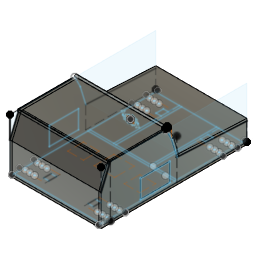
structure_vistech006_vigorini v10 (Autodesk Fusion 360 design; units mm, degrees)
Autodesk Fusion 360 part; units mm, degrees
note: some values were not read from the file. Set by a fixed rule: which face or edge a step refers to.
sketch "Sketch1" plane through (0, 0, 0) normal (0, 0, 1) x (1, 0, 0) in component "Base"
  line L0 (-125, -200) -> (125, -200)
  line L1 (125, -200) -> (125, 200)
  line L2 (125, 200) -> (-125, 200)
  line L3 (-125, 200) -> (-125, -200)
  line L4 (-125, -200) -> (125, 200) construction
  line L5 (125, -200) -> (-125, 200) construction
  dimension "d1" = 250
  dimension "d2" = 400
  constraint horizontal L0
  constraint perpendicular L0 L1
  constraint parallel L0 L2
  constraint parallel L1 L3
  constraint coincident L4 origin
  constraint coincident L5 origin
  measures "d1" distance of L1.end L2.end
  measures "d2" distance of L0.end L1.end
extrude "Extrude1" add sketch "Sketch1" along normal blind 6 makes body 1 in component "Base"
sketch "Sketch2" plane through (0, 0, 6) normal (0, 0, 1) x (-1, 0, 0) in component "Base"
  line L0 (125, -200) -> (125, 200)
  line L1 (125, 200) -> (-125, 200)
  line L2 (-125, 200) -> (-125, -200)
  line L3 (-125, -200) -> (125, -200)
  line L4 (-119, -194) -> (119, -194)
  line L5 (119, 194) -> (-119, 194)
  line L6 (-119, 194) -> (-119, -194)
  line L7 (119, 194) -> (119, -194)
  line L8 (-119, -194) -> (-119, -200)
  line L9 (119, -194) -> (119, -200)
  line L10 (-119, 194) -> (-119, 200)
  line L11 (119, 194) -> (119, 200)
  line L12 (-119, -194) -> (-119, -14) construction
  line L13 (-119, -14) -> (-119, 194) construction
  line L14 (-119, -14) -> (119, -14)
  line L15 (-93.6209, -8.2136) -> (-93.6209, -8) construction
  line L16 (-119, -8.2136) -> (119, -8.2136)
  line L17 (-48, -194) -> (-48, -14)
  line L18 (48, -194) -> (48, -14)
  line L19 (-125, -174) -> (-54, -174) construction
  line L20 (-54, -174) -> (-54, -164) construction
  line L21 (-54, -164) -> (-68.1, -164)
  line L22 (-68.1, -164) -> (-68.1, -144)
  line L23 (-68.1, -144) -> (-54, -144)
  line L24 (-54, -144) -> (-54, -134) construction
  line L25 (-54, -134) -> (-125, -134) construction
  line L26 (-54, -194) -> (-54, -14)
  line L27 (125, -174) -> (54, -174) construction
  line L28 (54, -174) -> (54, -164) construction
  line L29 (54, -164) -> (68.1, -164)
  line L30 (68.1, -164) -> (68.1, -144)
  line L31 (68.1, -144) -> (54, -144)
  line L32 (54, -144) -> (54, -134) construction
  line L33 (54, -134) -> (125, -134) construction
  line L34 (54.2628, -194) -> (54.2628, -14)
  line L35 (125, 174) -> (54, 174) construction
  line L36 (54, 174) -> (54, 164) construction
  line L37 (54, 164) -> (68.1, 164)
  line L38 (68.1, 164) -> (68.1, 144)
  line L39 (68.1, 144) -> (54, 144)
  line L40 (54, 144) -> (54, 134) construction
  line L41 (54, 134) -> (125, 134) construction
  line L42 (-125, 174) -> (-54, 174) construction
  line L43 (-54, 174) -> (-54, 164) construction
  line L44 (-54, 164) -> (-68.1, 164)
  line L45 (-68.1, 164) -> (-68.1, 144)
  line L46 (-68.1, 144) -> (-54, 144)
  line L47 (-54, 144) -> (-54, 134) construction
  line L48 (-54, 134) -> (-125, 134) construction
  circle A0 centre (-112.12, -137.2) radius 1.5
  circle A1 centre (-99.32, -137.2) radius 1.5
  circle A2 centre (-86.52, -137.2) radius 1.5
  circle A3 centre (-112.2, -170.8) radius 1.5
  circle A4 centre (-99.4, -170.8) radius 1.5
  circle A5 centre (-86.6, -170.8) radius 1.5
  circle A6 centre (112.2, -137.2) radius 1.5
  circle A7 centre (99.4, -137.2) radius 1.5
  circle A8 centre (86.6, -137.2) radius 1.5
  circle A9 centre (86.6, -170.8) radius 1.5
  circle A10 centre (112.2, -170.8) radius 1.5
  circle A11 centre (99.4, -170.8) radius 1.5
  circle A12 centre (-112.2, 137.2) radius 1.5
  circle A13 centre (-99.4, 137.2) radius 1.5
  circle A14 centre (-86.6, 137.2) radius 1.5
  circle A15 centre (-112.2, 170.8) radius 1.5
  circle A16 centre (-99.4, 170.8) radius 1.5
  circle A17 centre (-86.6, 170.8) radius 1.5
  circle A18 centre (112.2, 170.8) radius 1.5
  circle A19 centre (99.4, 170.8) radius 1.5
  circle A20 centre (86.6, 170.8) radius 1.5
  circle A21 centre (112.2, 137.2) radius 1.5
  circle A22 centre (99.4, 137.2) radius 1.5
  circle A23 centre (86.6, 137.2) radius 1.5
  line L49 (54, 144) -> (54, 164)
  line L50 (-54, 144) -> (-54, 164)
  line L51 (28.025, 11.7864) -> (28.025, 65.8664) construction
  line L52 (28.025, 65.8664) -> (-28.025, 65.8664) construction
  line L53 (-28.025, 65.8664) -> (-28.025, 61.3869) construction
  line L54 (-28.025, 61.3869) -> (-28.025, 11.7864) construction
  line L55 (-28.025, 11.7864) -> (28.025, 11.7864) construction
  line L56 (-99, 24.3105) -> (-56, 24.3105) construction
  line L57 (-56, 24.3105) -> (-56, 67.5105) construction
  line L58 (-56, 67.5105) -> (-99, 67.5105) construction
  line L59 (-99, 67.5105) -> (-99, 24.3105) construction
  line L60 (99, 24.3105) -> (99, 67.5105) construction
  line L61 (99, 67.5105) -> (56, 67.5105) construction
  line L62 (56, 67.5105) -> (56, 24.3105) construction
  line L63 (56, 24.3105) -> (99, 24.3105) construction
  dimension "d9" = 388
  dimension "d10" = 238
  dimension "d11" = 180
  dimension "d14" = 202.2136
  dimension "d18" = 71
  dimension "d21" = 20
  dimension "d22" = 14.1
  dimension "d23" = 10
  dimension "d25" = 71
  dimension "d28" = 20
  dimension "d29" = 14.1
  dimension "d32" = 71
  dimension "d33" = 10
  dimension "d34" = 14.1
  dimension "d35" = 20
  dimension "d39" = 71
  dimension "d40" = 10
  dimension "d41" = 14.1
  dimension "d42" = 20
  dimension "d53" = 12.8
  dimension "d54" = 12.8
  dimension "d58" = 3
  dimension "d59" = 3
  dimension "d60" = 3
  dimension "d61" = 3
  dimension "d62" = 3
  dimension "d63" = 3
  dimension "d68" = 12.8
  dimension "d70" = 3
  dimension "d71" = 3
  dimension "d72" = 3
  dimension "d73" = 3
  dimension "d74" = 3
  dimension "d75" = 3
  dimension "d79" = 12.8
  dimension "d80" = 12.8
  dimension "d85" = 3
  dimension "d86" = 3
  dimension "d87" = 3
  dimension "d88" = 3
  dimension "d89" = 3
  dimension "d90" = 3
  dimension "d94" = 12.8
  dimension "d95" = 12.8
  dimension "d100" = 3
  dimension "d101" = 3
  dimension "d102" = 3
  dimension "d109" = 12.8
  dimension "d110" = 3
  dimension "d111" = 3
  dimension "d112" = 3
  dimension "d115" = 54.08
  dimension "d116" = 56.05
  dimension "d118" = 43
  dimension "d119" = 43.2
  dimension "d121" = 43.2
  dimension "d122" = 43
  constraint perpendicular L0 L4
  constraint perpendicular L2 L5
  constraint perpendicular L3 L6
  constraint perpendicular L3 L7
  constraint coincident L3 L8.end
  constraint perpendicular L3 L8
  constraint coincident L3 L9.end
  constraint perpendicular L3 L9
  constraint coincident L1 L10.end
  constraint perpendicular L1 L10
  constraint coincident L1 L11.end
  constraint perpendicular L1 L11
  constraint perpendicular L4 L12
  constraint perpendicular L5 L13
  constraint coincident L7 L14.end
  constraint perpendicular L7 L14
  constraint perpendicular L14 L15
  constraint coincident L6 L16.start
  constraint coincident L7 L16.end
  constraint perpendicular L7 L16
  constraint coincident L16 L15.start
  constraint coincident L4 L17.start
  constraint coincident L14 L17.end
  constraint perpendicular L14 L17
  constraint coincident L4 L18.start
  constraint coincident L14 L18.end
  constraint perpendicular L14 L18
  constraint coincident L2 L19.start
  constraint perpendicular L2 L19
  constraint perpendicular L19 L20
  constraint perpendicular L20 L21
  constraint perpendicular L21 L22
  constraint perpendicular L22 L23
  constraint perpendicular L23 L24
  constraint coincident L2 L25.end
  constraint perpendicular L2 L25
  constraint coincident L4 L26.start
  constraint perpendicular L14 L26
  constraint coincident L0 L27.start
  constraint perpendicular L7 L27
  constraint perpendicular L27 L28
  constraint perpendicular L28 L29
  constraint perpendicular L29 L30
  constraint perpendicular L30 L31
  constraint perpendicular L31 L32
  constraint coincident L0 L33.end
  constraint perpendicular L0 L33
  constraint coincident L4 L34.start
  constraint coincident L14 L34.end
  constraint perpendicular L14 L34
  constraint coincident L0 L35.start
  constraint perpendicular L34 L35
  constraint perpendicular L35 L36
  constraint perpendicular L34 L37
  constraint perpendicular L16 L38
  constraint perpendicular L38 L39
  constraint perpendicular L39 L40
  constraint coincident L0 L41.end
  constraint perpendicular L0 L41
  constraint coincident L2 L42.start
  constraint perpendicular L13 L42
  constraint perpendicular L42 L43
  constraint perpendicular L43 L44
  constraint perpendicular L44 L45
  constraint perpendicular L45 L46
  constraint perpendicular L46 L47
  constraint coincident L2 L48.end
  constraint perpendicular L2 L48
  constraint perpendicular L37 L49
  constraint perpendicular L44 L50
  constraint perpendicular L51 L52
  constraint perpendicular L52 L53
  constraint perpendicular L52 L54
  constraint perpendicular L51 L55
  constraint perpendicular L56 L57
  constraint perpendicular L56 L59
  constraint perpendicular L60 L61
  constraint perpendicular L61 L62
  constraint perpendicular L60 L63
  measures "d9" distance of L4.start L5.end
  measures "d10" distance of L5.start L5.end
  measures "d11" distance of L4.start L12.end
  measures "d14" distance of L5.end L16.start
  measures "d18" distance of L19.start L19.end
  measures "d21" distance of L21.end L22.end
  measures "d22" distance of L22.end L23.end
  measures "d23" distance of L23.end L24.end
  measures "d25" distance of L27.start L27.end
  measures "d28" distance of L29.end L30.end
  measures "d29" distance of L30.end L31.end
  measures "d32" distance of L35.start L35.end
  measures "d33" distance of L35.end L36.end
  measures "d34" distance of L36.end L37.end
  measures "d35" distance of L37.end L38.end
  measures "d39" distance of L42.start L42.end
  measures "d40" distance of L42.end L43.end
  measures "d41" distance of L43.end L44.end
  measures "d42" distance of L44.end L45.end
  measures "d53" distance of A0.centre A1.centre
  measures "d54" distance of A1.centre A2.centre
  measures "d58" diameter of A0
  measures "d59" diameter of A1
  measures "d60" diameter of A2
  measures "d61" diameter of A3
  measures "d62" diameter of A4
  measures "d63" diameter of A5
  measures "d68" distance of A7.centre A8.centre
  measures "d70" diameter of A8
  measures "d71" diameter of A7
  measures "d72" diameter of A6
  measures "d73" diameter of A9
  measures "d74" diameter of A11
  measures "d75" diameter of A10
  measures "d79" distance of A15.centre A16.centre
  measures "d80" distance of A16.centre A17.centre
  measures "d85" diameter of A12
  measures "d86" diameter of A13
  measures "d87" diameter of A14
  measures "d88" diameter of A15
  measures "d89" diameter of A16
  measures "d90" diameter of A17
  measures "d94" distance of A18.centre A19.centre
  measures "d95" distance of A19.centre A20.centre
  measures "d100" diameter of A20
  measures "d101" diameter of A19
  measures "d102" diameter of A18
  measures "d109" distance of A22.centre A23.centre
  measures "d110" diameter of A23
  measures "d111" diameter of A22
  measures "d112" diameter of A21
  measures "d115" distance of L51.start L51.end
  measures "d116" distance of L51.end L52.end
  measures "d118" distance of L56.start L56.end
  measures "d119" distance of L56.end L57.end
  measures "d121" distance of L60.start L60.end
  measures "d122" distance of L60.end L61.end
extrude "Extrude2" cut sketch "Sketch2" along normal through all and the other way through all contours L29 L30 L31 L34 | L21 L22 L23 L26 | L37 L38 L39 L49 | L44 L45 L46 L50 | A0 | A1 | A2 | A3 | A4 | A5 | A6 | A7 | A8 | A9 | A10 | A11 | A12 | A13 | A14 | A15 | A16 | A17 | A18 | A19 | A20 | A21 | A22 | A23 bodies 1 in component "Base"
sketch "Sketch2 (2)" plane through (0, 0, 6) normal (0, 0, 1) x (-1, 0, 0) in component "Right_panel"
extrude "Extrude1'" add sketch "Sketch2" along normal blind 140 separate body contours L1 L2 L3 L6 L8 L10 makes body 2 in component "Right_panel"
sketch "Sketch3" plane through (125, 0, 0) normal (1, 0, 0) x (0, 1, 0) in component "Right_panel"
  line L0 (-200, 6) -> (200, 6)
  line L1 (200, 6) -> (200, 146)
  line L2 (200, 146) -> (-200, 146)
  line L3 (-200, 146) -> (-200, 6)
  line L4 (200, 6) -> (200, 56) construction
  line L5 (200, 6) -> (8, 6) construction
  line L6 (8, 6) -> (8, 66) construction
  line L7 (8, 66) -> (8, 116) construction
  line L8 (8, 66) -> (200, 56)
  line L9 (-7, 116) -> (8, 66)
  line L10 (-7, 116) -> (-22, 146)
  line L11 (-7, 116) -> (-7, 146) construction
  line L12 (-7, 146) -> (-22, 146) construction
  line L13 (-200, 146) -> (-200, 86) construction
  line L14 (-200, 146) -> (-175, 146) construction
  line L15 (-200, 86) -> (-175, 146)
  line L16 (-12, 66) -> (-92, 66)
  line L17 (-92, 66) -> (-92, 16)
  line L18 (-92, 16) -> (-12, 16)
  line L19 (-12, 16) -> (-12, 66)
  line L20 (-175, 146) -> (-175, 6) construction
  dimension "d152" = 50
  dimension "d153" = 192
  dimension "d155" = 60
  dimension "d156" = 50
  dimension "d157" = 15
  dimension "d159" = 30
  dimension "d160" = 15
  dimension "d161" = 60
  dimension "d162" = 25
  dimension "d164" = 20
  dimension "d165" = 80
  dimension "d166" = 50
  dimension "d167" = 140
  constraint coincident L0.end L1.start
  constraint perpendicular L0 L4
  constraint perpendicular L1 L5
  constraint perpendicular L5 L6
  constraint parallel L6 L7
  constraint coincident L2 L10.end
  constraint perpendicular L2 L11
  constraint perpendicular L11 L12
  constraint coincident L2.end L3.start
  constraint perpendicular L2 L13
  constraint perpendicular L3 L14
  constraint perpendicular L16 L17
  constraint perpendicular L17 L18
  constraint perpendicular L16 L19
  constraint perpendicular L0 L20
  measures "d152" distance of L0.end L4.end
  measures "d153" distance of L0.end L5.end
  measures "d155" distance of L5.end L6.end
  measures "d156" distance of L6.end L7.end
  measures "d157" distance of L7.end L9.start
  measures "d159" distance of L9.start L11.end
  measures "d160" distance of L11.end L10.end
  measures "d161" distance of L2.end L13.end
  measures "d162" distance of L2.end L14.end
  measures "d164" distance of L6.end L16.start
  measures "d165" distance of L16.start L16.end
  measures "d166" distance of L16.end L17.end
  measures "d167" distance of L14.end L20.end
extrude "Extrude2'" cut sketch "Sketch3" against normal through all contours L2 L3 L15 | L1 L2 L8 L9 L10 bodies 2 in component "Right_panel"
sketch "Sketch1 (2)" plane through (0, 0, 6) normal (0, 0, 1) x (-1, 0, 0) in component "left_panel"
extrude "Extrude1''" add sketch "Sketch2" along normal blind 140 separate body contours L0 L1 L3 L7 L9 L11 makes body 3 in component "left_panel"
sketch "Sketch2 (3)" plane through (-125, 0, 0) normal (-1, 0, 0) x (0, -1, 0) in component "left_panel"
  line L0 (-200, 6) -> (200, 6)
  line L1 (200, 6) -> (200, 146)
  line L2 (200, 146) -> (-200, 146)
  line L3 (-200, 146) -> (-200, 6)
  line L4 (-200, 6) -> (-8, 6) construction
  line L5 (-200, 6) -> (-200, 56) construction
  line L6 (-8, 6) -> (-8, 66) construction
  line L7 (-8, 66) -> (7, 116)
  line L8 (7, 116) -> (22, 146)
  line L9 (-8, 66) -> (-200, 56)
  line L10 (12, 66) -> (92, 66)
  line L11 (92, 66) -> (92, 16)
  line L12 (92, 16) -> (12, 16)
  line L13 (12, 16) -> (12, 66)
  line L14 (200, 146) -> (175, 146) construction
  line L15 (200, 146) -> (200, 86)
  line L16 (175, 146) -> (200, 86)
  dimension "d170" = 192
  dimension "d171" = 50
  dimension "d172" = 60
  dimension "d177" = 80
  dimension "d178" = 50
  dimension "d180" = 25
  dimension "d181" = 60
  constraint coincident L0.start L3.end
  constraint perpendicular L3 L4
  constraint perpendicular L4 L5
  constraint perpendicular L4 L6
  constraint perpendicular L10 L11
  constraint perpendicular L11 L12
  constraint coincident L1.end L2.start
  constraint perpendicular L1 L14
  constraint perpendicular L14 L15
  measures "d170" distance of L0.start L4.end
  measures "d171" distance of L0.start L5.end
  measures "d172" distance of L4.end L6.end
  measures "d177" distance of L10.start L10.end
  measures "d178" distance of L10.end L11.end
  measures "d180" distance of L1.end L14.end
  measures "d181" distance of L1.end L15.end
extrude "Extrude2''" cut sketch "Sketch2 (3)" against normal through all contours L2 L3 L7 L8 L9 | L1 L2 L15 L16 bodies 3 in component "left_panel"
extrude "Extrude4" cut sketch "Sketch2 (3)" against normal up to surface (6 mm away) contours L10 L11 L12 L13 bodies 3 in component "left_panel"
extrude "Extrude4'" cut sketch "Sketch3" against normal up to surface (6 mm away) contours L16 L17 L18 L19 bodies 2 in component "Right_panel"
sketch "Sketch1 (3)" plane through (125, 0, 0) normal (1, 0, 0) x (0, 1, 0) in component "Right_driver_panel"
extrude "Extrude1'''" add sketch "Sketch3" against normal up to surface (6 mm away) separate body contours L16 L17 L18 L19 makes body 4 in component "Right_driver_panel"
sketch "Sketch1 (4)" plane through (-125, 0, 0) normal (-1, 0, 0) x (0, -1, 0) in component "Left_driver_panel"
extrude "Extrude1''''" add sketch "Sketch2 (3)" against normal up to surface (6 mm away) separate body contours L10 L11 L12 L13 makes body 5 in component "Left_driver_panel"
sketch "Sketch1 (5)" plane through (0, 0, 6) normal (0, 0, 1) x (-1, 0, 0) in component "Front_panel"
extrude "Extrude1'''''" add sketch "Sketch2" along normal blind 50 separate body contours L3 L4 L8 L9 makes body 6 in component "Front_panel"
sketch "Sketch1 (6)" plane through (0, 0, 6) normal (0, 0, 1) x (-1, 0, 0) in component "mid_panel"
extrude "Extrude1''''''" add sketch "Sketch2" along normal blind 60 separate body contours L6 L7 L14 L16 makes body 7 in component "mid_panel"
extrude "Extrude1'''''''" add sketch "Sketch2" along normal blind 80 separate body contours L1 L5 L10 L11 makes body 8 in component "Back_panel"
extrude "Extrude1''''''''" add sketch "Sketch2" along normal blind 60 separate body contours L4 L14 L17 L26 makes body 9 in component "Front_support_right_panel"
sketch "Sketch1 (7)" plane through (48, 0, 0) normal (-1, 0, 0) x (0, -1, 0) in component "Front_support_right_panel"
  line L0 (-194, 6) -> (-14, 6)
  line L1 (-14, 6) -> (-14, 66)
  line L2 (-14, 66) -> (-194, 66)
  line L3 (-194, 66) -> (-194, 6)
  line L4 (-194, 66) -> (-194, 56) construction
  line L5 (-194, 56) -> (-14, 66)
  dimension "d203" = 10
  constraint coincident L2.end L3.start
  constraint perpendicular L2 L4
  constraint coincident L1.end L2.start
  measures "d203" distance of L2.end L4.end
extrude "Extrude2'''" cut sketch "Sketch1 (7)" against normal up to surface (6 mm away) contours L2 L3 L5 bodies 9 in component "Front_support_right_panel"
extrude "Extrude1'''''''''" add sketch "Sketch2" along normal blind 60 separate body contours L4 L14 L18 L34 makes body 10 in component "Front_support_left_panel"
sketch "Sketch1 (8)" plane through (-54.2628, 0, 0) normal (-1, 0, 0) x (0, -1, 0) in component "Front_support_left_panel"
  line L0 (-194, 6) -> (-14, 6)
  line L1 (-14, 6) -> (-14, 66)
  line L2 (-14, 66) -> (-194, 66)
  line L3 (-194, 66) -> (-194, 6)
  line L4 (-194, 66) -> (-194, 56) construction
  line L5 (-194, 56) -> (-14, 66)
  dimension "d208" = 10
  constraint coincident L2.end L3.start
  constraint perpendicular L2 L4
  constraint coincident L1.end L2.start
  measures "d208" distance of L2.end L4.end
extrude "Extrude2''''" cut sketch "Sketch1 (8)" against normal up to surface (6.2628 mm away) contours L2 L3 L5 bodies 10 in component "Front_support_left_panel"
sketch "Sketch2 (4)" plane through (0, 0, 146) normal (0, 0, 1) x (-1, 0, 0) in component "Top_panel"
  line L0 (125, 175) -> (119, 175)
  line L1 (119, 175) -> (119, 22)
  line L2 (119, 22) -> (125, 22)
  line L3 (125, 22) -> (125, 175)
extrude "Extrude1''''''''''" add sketch "Sketch2 (4)" along normal blind 6 separate body makes body 11 in component "Top_panel"
move_face "OffsetFaces1" offset 244 1 faces at (-119, -124, 148) on bodies 11 in component "Top_panel"
sketch "Sketch1 (9)" plane through (-119, 0, 0) normal (1, 0, 0) x (0, 1, 0)
  line L0 (-12, 66) -> (-12, 16)
  line L1 (-12, 16) -> (-92, 16)
  line L2 (-92, 16) -> (-92, 66)
  line L3 (-92, 66) -> (-12, 66)
  line L4 (-175, 146) -> (-200, 86)
  line L5 (-200, 86) -> (-200, 6)
  line L6 (-200, 6) -> (200, 6)
  line L7 (200, 6) -> (200, 56)
  line L8 (200, 56) -> (8, 66)
  line L9 (8, 66) -> (-7, 116)
  line L10 (-7, 116) -> (-22, 146)
  line L11 (-22, 146) -> (-175, 146)
  line L12 (-200, 86) -> (-194, 86)
  line L13 (-194, 86) -> (-171.2617, 146)
  dimension "d214" = 6
  constraint coincident L4.end L5.start
  constraint perpendicular L5 L12
  constraint coincident L11 L13.end
  measures "d214" distance of L4.end L12.end
extrude "Extrude1'''''''''''" add sketch "Sketch1 (9)" along normal up to surface (238 mm away) separate body contours L4 L11 L12 L13 makes body 12 in component "support_back_panel"
sketch "Sketch1 (10)" plane through (0, 3.4498, 66.237) normal (0, 0.052013, 0.998646) x (-1, 0, 0) in component "Front_top_panel"
  line L0 (-119, -196.8166) -> (-119, -4.5563)
  line L1 (-119, -4.5563) -> (-125, -4.5563)
  line L2 (-125, -4.5563) -> (-125, -196.8166)
  line L3 (-125, -196.8166) -> (-119, -196.8166)
extrude "Extrude1''''''''''''" add sketch "Sketch1 (10)" along normal blind 6 separate body makes body 13 in component "Front_top_panel"
move_face "OffsetFaces1'" offset 244 1 faces at (119, 72.2081, 66.6613) on bodies 13 in component "Front_top_panel"
move_face "OffsetFaces2" offset 2.2 1 faces at (41.6667, 8.2081, 69.9946) on bodies 13 in component "Front_top_panel"
sketch "Sketch2 (5)" plane through (0, 25.5046, 7.6514) normal (0, 0.957826, 0.287348) x (-1, 0, 0) in component "window_lower_panel"
  line L0 (-119, 60.9178) -> (-119, 113.1193)
  line L1 (-119, 113.1193) -> (-125, 113.1193)
  line L2 (-125, 113.1193) -> (-125, 60.9178)
  line L3 (-125, 60.9178) -> (-119, 60.9178)
extrude "Extrude1'''''''''''''" add sketch "Sketch2 (5)" along normal blind 6 separate body makes body 14 in component "window_lower_panel"
move_face "OffsetFaces1''" offset 244 1 faces at (119, 4.9157, 83.2414) on bodies 14 in component "window_lower_panel"
sketch "Sketch1 (11)" plane through (0, 40.8, 20.4) normal (0, 0.894427, 0.447214) x (-1, 0, 0) in component "window_upper_panel"
  line L0 (-119, 106.884) -> (-119, 140.4251)
  line L1 (-119, 140.4251) -> (-125, 140.4251)
  line L2 (-125, 140.4251) -> (-125, 106.884)
  line L3 (-125, 106.884) -> (-119, 106.884)
extrude "Extrude1''''''''''''''" add sketch "Sketch1 (11)" along normal blind 6 separate body makes body 15 in component "window_upper_panel"
move_face "OffsetFaces1'''" offset 244 1 faces at (119, -13.4223, 137.7889) on bodies 15 in component "window_upper_panel"
move_face "OffsetFaces2'" offset 5.4 1 faces at (-41.6667, -22, 150) on bodies 11 in component "Top_panel"
move_face "OffsetFaces2''" offset 4 1 faces at (-41.6667, -20.2111, 146.8944) on bodies 15 in component "window_upper_panel"
sketch "Sketch2 (6)" plane through (125, 0, 0) normal (1, 0, 0) x (0, 1, 0) in component "window_upper_panel"
  line L0 (-23.7889, 149.5777) -> (-7, 116)
  line L1 (-7, 116) -> (-1.6334, 118.6833)
  line L2 (-1.6334, 118.6833) -> (-18.4223, 152.261)
  line L3 (-18.4223, 152.261) -> (-23.7889, 149.5777)
  line L4 (-18.4223, 152.261) -> (-18.2915, 151.9995)
  line L5 (-18.9454, 151.9995) -> (-18.4223, 152.261)
  line L6 (-18.9454, 151.9995) -> (-18.2915, 151.9995)
  constraint coincident L2.end L3.start
  constraint coincident L2 L4.end
  constraint perpendicular L3 L4
  constraint coincident L3 L5.start
  constraint perpendicular L4 L5
  constraint horizontal L6
extrude "Extrude2'''''" cut sketch "Sketch2 (6)" against normal up to surface (250 mm away) contours L2 L3 L4 L5 L6 bodies 11 in component "Top_panel"
extrude "Extrude2''''''" cut sketch "Sketch2 (6)" against normal up to surface (250 mm away) contours L2 L3 L4 L5 L6 bodies 15 in component "window_upper_panel"
sketch "Sketch3 (2)" plane through (-125, 0, 0) normal (-1, 0, 0) x (0, -1, 0) in component "Top_panel"
  line L0 (18.2915, 151.9995) -> (18.2918, 152)
  line L1 (18.2918, 152) -> (16.6, 152)
  line L2 (16.6, 152) -> (16.6, 146)
  line L3 (16.6, 146) -> (175, 146)
  line L4 (175, 146) -> (175, 152)
  line L5 (175, 152) -> (18.9443, 152)
  line L6 (18.9443, 152) -> (18.9454, 151.9995)
  line L7 (18.9454, 151.9995) -> (18.2915, 151.9995)
  line L8 (16.6, 152) -> (18.2918, 152)
  line L9 (18.2918, 152) -> (16.6, 148.6162)
  line L10 (16.6, 148.6162) -> (16.6, 152)
  constraint coincident L1.end L2.start
  constraint coincident L0.end L1.start
  constraint coincident L2 L9.end
  constraint perpendicular L1 L10
extrude "Extrude3" cut sketch "Sketch3 (2)" against normal up to surface (250 mm away) contours L0 L1 L2 L8 L9 L10 bodies 11 in component "Top_panel"
extrude "Extrude3'" cut sketch "Sketch3 (2)" against normal up to surface (250 mm away) contours L1 L2 L8 L9 L10 bodies 15 in component "window_upper_panel"
sketch "Sketch3 (3)" plane through (125, 0, 0) normal (1, 0, 0) x (0, 1, 0) in component "window_upper_panel"
  line L0 (-16.6, 148.6164) -> (-16.6, 148.6162)
  line L1 (-16.6, 148.6162) -> (-18.2915, 151.9995)
  line L2 (-18.2915, 151.9995) -> (-18.9454, 151.9995)
  line L3 (-18.9454, 151.9995) -> (-23.7889, 149.5777)
  line L4 (-23.7889, 149.5777) -> (-7, 116)
  line L5 (-7, 116) -> (-1.6334, 118.6833)
  line L6 (-1.6334, 118.6833) -> (-16.6, 148.6164)
  line L7 (-18.9454, 151.9995) -> (-23.7889, 149.5777)
  line L8 (-23.7889, 149.5777) -> (-21.9999, 145.9999)
  line L9 (-21.9999, 145.9999) -> (-16.6, 145.9999)
  line L10 (-16.6, 145.9999) -> (-16.6, 148.6164)
  line L11 (-16.6, 148.6164) -> (-18.2915, 151.9995)
  line L12 (-18.2915, 151.9995) -> (-18.9454, 151.9995)
  constraint coincident L2.end L3.start
  constraint coincident L3.end L4.start
  constraint coincident L4 L8.end
  constraint perpendicular L3 L8
  constraint horizontal L9
  constraint coincident L0.start L6.end
  constraint coincident L1.end L2.start
sketch "Sketch2 (7)" plane through (0, 31.2515, 9.3755) normal (0, 0.957826, 0.287348) x (-1, 0, 0)
  line L0 (-125, 60.9178) -> (125, 60.9178)
  line L1 (125, 60.9178) -> (125, 113.1193)
  line L2 (125, 113.1193) -> (-125, 113.1193)
  line L3 (-125, 113.1193) -> (-125, 60.9178)
  line L4 (10.3875, 71.1385) -> (20.7751, 77.1357) construction
  line L5 (20.7751, 77.1357) -> (20.7751, 101.1247) construction
  line L6 (20.7751, 101.1247) -> (10.3875, 107.122) construction
  line L7 (-10.3875, 107.122) -> (-20.7751, 101.1247) construction
  line L8 (-20.7751, 101.1247) -> (-20.7751, 77.1357) construction
  line L9 (-20.7751, 77.1357) -> (-10.3875, 71.1385) construction
  line L10 (-20.7751, 89.1302) -> (-10.3875, 71.1385) construction
  line L11 (10.3875, 71.1385) -> (20.7751, 89.1302) construction
  line L12 (20.7751, 89.1302) -> (10.3875, 107.122) construction
  line L13 (-10.3875, 107.122) -> (-20.7751, 89.1302) construction
  line L14 (-7.7907, 75.6364) -> (0, 71.1385) construction
  line L15 (0, 71.1385) -> (7.7907, 75.6364) construction
  line L16 (-11.686, 95.8771) -> (-15.5813, 89.1302) construction
  line L17 (-15.5813, 89.1302) -> (-11.686, 82.3833) construction
  line L18 (-7.7907, 75.6364) -> (7.7907, 75.6364) construction
  line L19 (7.7907, 75.6364) -> (15.5813, 89.1302) construction
  line L20 (15.5813, 89.1302) -> (11.686, 95.8771) construction
  line L21 (0, 102.6241) -> (-11.686, 95.8771) construction
  line L22 (-11.686, 95.8771) -> (-11.686, 82.3833) construction
  line L23 (-11.686, 82.3833) -> (0, 75.6364) construction
  line L24 (0, 75.6364) -> (11.686, 82.3833) construction
  line L25 (11.686, 82.3833) -> (11.686, 95.8771) construction
  line L26 (11.686, 95.8771) -> (0, 102.6241) construction
  line L27 (5.843, 99.2506) -> (-5.843, 99.2506) construction
  line L28 (-5.843, 99.2506) -> (-11.686, 89.1302) construction
  line L29 (-11.686, 89.1302) -> (-5.843, 79.0099) construction
  line L30 (-5.843, 79.0099) -> (5.843, 79.0099) construction
  line L31 (5.843, 79.0099) -> (11.686, 89.1302) construction
  line L32 (11.686, 89.1302) -> (5.843, 99.2506) construction
  line L33 (8.7645, 94.1904) -> (0, 99.2506) construction
  line L34 (0, 99.2506) -> (-8.7645, 94.1904) construction
  line L35 (-8.7645, 94.1904) -> (-8.7645, 84.0701) construction
  line L36 (-8.7645, 84.0701) -> (0, 79.0099) construction
  line L37 (0, 79.0099) -> (8.7645, 84.0701) construction
  line L38 (8.7645, 84.0701) -> (8.7645, 94.1904) construction
  line L39 (8.7645, 89.1302) -> (4.3822, 96.7205) construction
  line L40 (4.3822, 96.7205) -> (-4.3822, 96.7205) construction
  line L41 (-4.3822, 96.7205) -> (-8.7645, 89.1302) construction
  line L42 (-8.7645, 89.1302) -> (-4.3822, 81.54) construction
  line L43 (-4.3822, 81.54) -> (4.3822, 81.54) construction
  line L44 (4.3822, 81.54) -> (8.7645, 89.1302) construction
  line L45 (6.5734, 85.3351) -> (6.5734, 92.9254) construction
  line L46 (6.5734, 92.9254) -> (0, 96.7205) construction
  line L47 (0, 96.7205) -> (-6.5734, 92.9254) construction
  line L48 (-6.5734, 92.9254) -> (-6.5734, 85.3351) construction
  line L49 (-6.5734, 85.3351) -> (0, 81.54) construction
  line L50 (0, 81.54) -> (6.5734, 85.3351) construction
  line L51 (-20.7751, 89.1302) -> (-20.7751, 101.1247)
  line L52 (-20.7751, 101.1247) -> (-10.3875, 107.122)
  line L53 (-20.7751, 89.1302) -> (-10.3875, 107.122)
  line L54 (10.3875, 107.122) -> (20.7751, 101.1247)
  line L55 (20.7751, 101.1247) -> (20.7751, 89.1302)
  line L56 (20.7751, 89.1302) -> (10.3875, 107.122)
  line L57 (-20.7751, 89.1302) -> (-10.3875, 71.1385)
  line L58 (-10.3875, 71.1385) -> (-20.7751, 77.1357)
  line L59 (-20.7751, 77.1357) -> (-20.7751, 89.1302)
  line L60 (10.3875, 71.1385) -> (20.7751, 77.1357)
  line L61 (20.7751, 77.1357) -> (20.7751, 89.1302)
  line L62 (10.3875, 71.1385) -> (20.7751, 89.1302)
  line L63 (0, 71.1385) -> (-7.7907, 75.6364)
  line L64 (-7.7907, 75.6364) -> (7.7907, 75.6364)
  line L65 (0, 71.1385) -> (7.7907, 75.6364)
  line L66 (-15.5813, 89.1302) -> (-11.686, 82.3833)
  line L67 (-15.5813, 89.1302) -> (-11.686, 95.8771)
  line L68 (-11.686, 95.8771) -> (-11.686, 82.3833)
  line L69 (15.5813, 89.1302) -> (11.686, 82.3833)
  line L70 (11.686, 95.8771) -> (11.686, 82.3833)
  line L71 (11.686, 95.8771) -> (15.5813, 89.1302)
  line L72 (-5.843, 99.2506) -> (5.843, 99.2506)
  line L73 (-5.843, 99.2506) -> (0, 102.6241)
  line L74 (0, 102.6241) -> (5.843, 99.2506)
  point P0 (0, 89.1302)
  point P1 (0, 89.1302)
  point P2 (0, 89.1302)
  point P3 (0, 89.1302)
  point P4 (0, 89.1302)
  point P5 (0, 89.1302)
  point P6 (0, 89.1302)
  point P7 (0, 89.1302)
  point P8 (0, 89.1302)
  constraint midpoint L8 L10.start
  constraint coincident P8 P7
  constraint midpoint L26 L27.start
  constraint midpoint L32 L33.start
  constraint midpoint L38 L39.start
  constraint midpoint L44 L45.start
  constraint vertical L68
sketch "Sketch3 (4)" plane through (0, 31.2515, 9.3755) normal (0, 0.957826, 0.287348) x (-1, 0, 0) in component "window_lower_panel"
extrude "Extrude3''" [suppressed] in component "Right_panel"
extrude "Extrude3'''" [suppressed] in component "left_panel"
component "Base" placed x (1, 0, 0) y (0, 1, 0) z (0, 0, 1) at (0, 0, 0)
component "Right_panel" placed x (1, 0, 0) y (0, 1, 0) z (0, 0, 1) at (0, 0, 0)
component "left_panel" placed x (1, 0, 0) y (0, 1, 0) z (0, 0, 1) at (0, 0, 0)
component "Right_driver_panel" placed x (1, 0, 0) y (0, 1, 0) z (0, 0, 1) at (0, 0, 0)
component "Left_driver_panel" placed x (1, 0, 0) y (0, 1, 0) z (0, 0, 1) at (0, 0, 0)
component "Front_panel" placed x (1, 0, 0) y (0, 1, 0) z (0, 0, 1) at (0, 0, 0)
component "mid_panel" placed x (1, 0, 0) y (0, 1, 0) z (0, 0, 1) at (0, 0, 0)
component "Back_panel" placed x (1, 0, 0) y (0, 1, 0) z (0, 0, 1) at (0, 0, 0)
component "Front_support_right_panel" placed x (1, 0, 0) y (0, 1, 0) z (0, 0, 1) at (0, 0, 0)
component "Front_support_left_panel" placed x (1, 0, 0) y (0, 1, 0) z (0, 0, 1) at (0, 0, 0)
component "Top_panel" placed x (1, 0, 0) y (0, 1, 0) z (0, 0, 1) at (-2.4744, -1.6524, -6.0704)
component "support_back_panel" placed x (1, 0, 0) y (0, 1, 0) z (0, 0, 1) at (0, 0, 0)
component "Front_top_panel" placed x (1, 0, 0) y (0, 1, 0) z (0, 0, 1) at (0, 0, 0)
component "window_lower_panel" placed x (1, 0, 0) y (0, 1, 0) z (0, 0, 1) at (0, 0, 0)
component "window_upper_panel" placed x (1, 0, 0) y (0, 1, 0) z (0, 0, 1) at (0, 0, 0)
